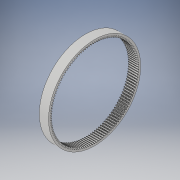
# Autodesk Inventor part: Component 21 (Hollow Wheel)
Saved by Autodesk Inventor 2018 (Build 220112000, 112)
## iProperties
Created: 2023-03-18
Part Number: Component 21 (Hollow Wheel)
Material: Generic
Document SubType Name: Modeling
Designer: Habib Mohamed
Density: 1 g/cm^3
Appearance: Default
Author: Habib Mohamed
Autodesk Inventor part; units mm, degrees
(part 1 of 2)
ref_plane "YZ Plane" through (0, 0, 0) normal (1, 0, 0) x (0, 1, 0)
ref_plane "XZ Plane" through (0, 0, 0) normal (0, 1, 0) x (-1, 0, 0)
ref_plane "XY Plane" through (0, 0, 0) normal (0, 0, 1) x (1, 0, 0)
sketch "Sketch1" plane through (0, 0, 0) normal (1, 0, 0) x (0, 1, 0)
  circle A0 centre (0, 0) radius 35
  line L0 (0, 0) -> (50.8877, 0) construction
  arc A1 (33.5687, 0.2221) -> (32.568, 0.5633) centre (30.706, -6.5366) ccw
  arc A2 (33.6297, 0.1304) -> (33.5687, 0.2221) centre (33.5297, 0.13) ccw
  arc A3 (32.4933, 0.658) -> (32.568, 0.5633) centre (32.5933, 0.66) ccw
  arc A4 (32.568, -0.5633) -> (33.5687, -0.2221) centre (30.706, 6.5366) ccw
  arc A5 (33.5687, -0.2221) -> (33.6297, -0.1304) centre (33.5297, -0.13) ccw
  arc A6 (32.568, -0.5633) -> (32.4933, -0.658) centre (32.5933, -0.66) ccw
  arc A7 (32.4252, 2.2033) -> (32.5043, 2.1123) centre (32.525, 2.2101) ccw
  arc A8 (33.5413, 1.3754) -> (33.5979, 1.4699) centre (33.498, 1.4656) ccw
  arc A9 (32.5579, 0.987) -> (33.5413, 1.3754) centre (30.3602, 7.9903) ccw
  arc A10 (32.5579, 0.987) -> (32.4878, 0.8889) centre (32.5878, 0.8916) ccw
  arc A11 (33.5202, 1.8191) -> (32.5043, 2.1123) centre (30.9823, -5.0682) ccw
  arc A12 (33.5855, 1.7304) -> (33.5202, 1.8191) centre (33.4856, 1.7253) ccw
  arc A13 (32.2837, 3.7437) -> (32.3669, 3.6565) centre (32.383, 3.7552) ccw
  arc A14 (33.4379, 2.9698) -> (33.4899, 3.0669) centre (33.3903, 3.0578) ccw
  arc A15 (32.474, 2.5351) -> (33.4379, 2.9698) centre (29.9456, 9.4258) ccw
  arc A16 (32.474, 2.5351) -> (32.4088, 2.4337) centre (32.5085, 2.4412) ccw
  arc A17 (33.3956, 3.412) -> (32.3669, 3.6565) centre (31.1883, -3.5883) ccw
  arc A18 (33.4651, 3.3265) -> (33.3956, 3.412) centre (33.3656, 3.3166) ccw
  arc A19 (32.069, 5.2756) -> (32.1563, 5.1924) centre (32.1676, 5.2918) ccw
  arc A20 (33.2587, 4.5575) -> (33.306, 4.657) centre (33.207, 4.6431) ccw
  arc A21 (32.3166, 4.0774) -> (33.2587, 4.5575) centre (29.4632, 10.84) ccw
  arc A22 (32.3166, 4.0774) -> (32.2562, 3.973) centre (32.3555, 3.9852) ccw
  arc A23 (33.1955, 4.9972) -> (32.1563, 5.1924) centre (31.3237, -2.1002) ccw
  arc A24 (33.2689, 4.9151) -> (33.1955, 4.9972) centre (33.17, 4.9005) ccw
  arc A25 (31.7816, 6.7955) -> (31.8728, 6.7166) centre (31.8794, 6.8164) ccw
  arc A26 (33.0041, 6.1349) -> (33.0467, 6.2364) centre (32.9484, 6.2179) ccw
  arc A27 (32.086, 5.6104) -> (33.0041, 6.1349) centre (28.9141, 12.2297) ccw
  arc A28 (32.086, 5.6104) -> (32.0307, 5.5033) centre (32.1292, 5.5203) ccw
  arc A29 (32.9201, 6.571) -> (31.8728, 6.7166) centre (31.3882, -0.6074) ccw
  arc A30 (32.9973, 6.4925) -> (32.9201, 6.571) centre (32.8992, 6.4732) ccw
  arc A31 (31.4223, 8.3) -> (31.5171, 8.2256) centre (31.519, 8.3256) ccw
  arc A32 (32.6749, 7.6983) -> (32.7125, 7.8018) centre (32.6152, 7.7786) ccw
  arc A33 (31.7827, 7.1308) -> (32.6749, 7.6983) centre (28.2994, 13.5916) ccw
  arc A34 (31.7827, 7.1308) -> (31.7325, 7.0212) centre (31.8302, 7.0428) ccw
  arc A35 (32.5701, 8.13) -> (31.5171, 8.2256) centre (31.3815, 0.8868) ccw
  arc A36 (32.651, 8.0552) -> (32.5701, 8.13) centre (32.5539, 8.0313) ccw
  arc A37 (30.9918, 9.7858) -> (31.09, 9.7159) centre (31.0871, 9.8159) ccw
  arc A38 (32.2715, 9.2443) -> (32.3042, 9.3495) centre (32.2082, 9.3217) ccw
  arc A39 (31.4074, 8.635) -> (32.2715, 9.2443) centre (27.6206, 14.9228) ccw
  arc A40 (31.4074, 8.635) -> (31.3625, 8.5231) centre (31.459, 8.5493) ccw
  arc A41 (32.1464, 9.6705) -> (31.09, 9.7159) centre (31.3038, 2.379) ccw
  arc A42 (32.2308, 9.5997) -> (32.1464, 9.6705) centre (32.1349, 9.5712) ccw
  arc A43 (30.491, 11.2493) -> (30.5925, 11.1842) centre (30.5848, 11.2839) ccw
  arc A44 (31.7951, 10.7694) -> (31.8228, 10.876) centre (31.7282, 10.8437) ccw
  arc A45 (30.961, 10.1196) -> (31.7951, 10.7694) centre (26.8793, 16.2201) ccw
  arc A46 (30.961, 10.1196) -> (30.9214, 10.0057) centre (31.0166, 10.0365) ccw
  arc A47 (31.6499, 11.1891) -> (30.5925, 11.1842) centre (31.1551, 3.8658) ccw
  arc A48 (31.7375, 11.1224) -> (31.6499, 11.1891) centre (31.6431, 11.0894) ccw
  arc A49 (29.9212, 12.6874) -> (30.0257, 12.6272) centre (30.0133, 12.7264) ccw
  arc A50 (31.2467, 12.2701) -> (31.2692, 12.3779) centre (31.1763, 12.3411) ccw
  arc A51 (30.4444, 11.5814) -> (31.2467, 12.2701) centre (26.0771, 17.4807) ccw
  arc A52 (30.4444, 11.5814) -> (30.4103, 11.4657) centre (30.5039, 11.501) ccw
  arc A53 (31.0816, 12.6824) -> (30.0257, 12.6272) centre (30.9359, 5.3439) ccw
  arc A54 (31.1723, 12.62) -> (31.0816, 12.6824) centre (31.0796, 12.5824) ccw
  arc A55 (29.2836, 14.0967) -> (29.3909, 14.0416) centre (29.3738, 14.1401) ccw
  arc A56 (30.6275, 13.743) -> (30.6449, 13.8517) centre (30.5537, 13.8105) ccw
  arc A57 (29.8588, 13.0168) -> (30.6275, 13.743) centre (25.2158, 18.7017) ccw
  arc A58 (29.8588, 13.0168) -> (29.8303, 12.8997) centre (29.9221, 12.9394) ccw
  arc A59 (30.443, 14.147) -> (29.3909, 14.0416) centre (30.6466, 6.8098) ccw
  arc A60 (30.5365, 14.0889) -> (30.443, 14.147) centre (30.4457, 14.047) ccw
  arc A61 (28.5797, 15.4741) -> (28.6894, 15.4242) centre (28.6677, 15.5218) ccw
  arc A62 (29.9389, 15.1847) -> (29.9511, 15.2941) centre (29.862, 15.2487) ccw
  arc A63 (29.2057, 14.4228) -> (29.9389, 15.1847) centre (24.2973, 19.8803) ccw
  arc A64 (29.2057, 14.4228) -> (29.1827, 14.3045) centre (29.2725, 14.3485) ccw
  arc A65 (29.7353, 15.5795) -> (28.6894, 15.4242) centre (30.2879, 8.2603) ccw
  arc A66 (29.8316, 15.5259) -> (29.7353, 15.5795) centre (29.7429, 15.4798) ccw
  arc A67 (27.8111, 16.8165) -> (27.923, 16.7718) centre (27.8966, 16.8682) ccw
  arc A68 (29.1824, 16.592) -> (29.1894, 16.702) centre (29.1026, 16.6523) ccw
  arc A69 (28.4863, 15.7962) -> (29.1824, 16.592) centre (23.3239, 21.0139) ccw
  arc A70 (28.4863, 15.7962) -> (28.469, 15.6768) centre (28.5566, 15.7251) ccw
  arc A71 (28.9603, 16.9767) -> (27.923, 16.7718) centre (29.8605, 9.6921) ccw
  arc A72 (29.059, 16.9278) -> (28.9603, 16.9767) centre (28.9726, 16.8775) ccw
  arc A73 (26.9794, 18.1207) -> (27.0934, 18.0814) centre (27.0624, 18.1765) ccw
  arc A74 (28.3599, 17.9618) -> (28.3616, 18.0719) centre (28.2773, 18.0182) ccw
  arc A75 (27.7024, 17.1337) -> (28.3599, 17.9618) centre (22.2976, 22.0999) ccw
  arc A76 (27.7024, 17.1337) -> (27.6909, 17.0137) centre (27.7761, 17.0661) ccw
  arc A77 (28.1198, 18.3355) -> (27.0934, 18.0814) centre (29.3655, 11.102) ccw
  arc A78 (28.2207, 18.2913) -> (28.1198, 18.3355) centre (28.1367, 18.2369) ccw
  arc A79 (26.0866, 19.384) -> (26.2023, 19.3501) centre (26.1669, 19.4436) ccw
  arc A80 (27.4731, 19.2909) -> (27.4696, 19.401) centre (27.3879, 19.3433) ccw
  arc A81 (26.8558, 18.4324) -> (27.4731, 19.2909) centre (21.2208, 23.1358) ccw
  arc A82 (26.8558, 18.4324) -> (26.85, 18.312) centre (26.9326, 18.3684) ccw
  arc A83 (27.2155, 19.6527) -> (26.2023, 19.3501) centre (28.804, 12.4866) ccw
  arc A84 (27.3184, 19.6134) -> (27.2155, 19.6527) centre (27.2371, 19.5551) ccw
  arc A85 (25.1348, 20.6033) -> (25.2519, 20.5749) centre (25.2121, 20.6666) ccw
  arc A86 (26.5241, 20.5763) -> (26.5154, 20.686) centre (26.4365, 20.6245) ccw
  arc A87 (25.9483, 19.6894) -> (26.5241, 20.5763) centre (20.0959, 24.1194) ccw
  arc A88 (25.9483, 19.6894) -> (25.9482, 19.5688) centre (26.0281, 19.6291) ccw
  arc A89 (26.2495, 20.9254) -> (25.2519, 20.5749) centre (28.1772, 13.8431) ccw
  arc A90 (26.3542, 20.891) -> (26.2495, 20.9254) centre (26.2758, 20.8289) ccw
  arc A91 (24.1259, 21.7759) -> (24.2444, 21.7532) centre (24.2002, 21.8429) ccw
  arc A92 (25.515, 21.815) -> (25.5011, 21.9243) centre (25.4252, 21.8591) ccw
  arc A93 (24.9821, 20.9018) -> (25.515, 21.815) centre (18.9255, 25.0482) ccw
  arc A94 (24.9821, 20.9018) -> (24.9877, 20.7813) centre (25.0646, 20.8453) ccw
  arc A95 (25.2241, 22.1507) -> (24.2444, 21.7532) centre (27.4867, 15.1681) ccw
  arc A96 (25.3303, 22.1213) -> (25.2241, 22.1507) centre (25.255, 22.0556) ccw
  arc A97 (23.0625, 22.8992) -> (23.1818, 22.8821) centre (23.1334, 22.9696) ccw
  arc A98 (24.4481, 23.0044) -> (24.429, 23.1128) centre (24.3563, 23.0441) ccw
  arc A99 (23.9592, 22.0668) -> (24.4481, 23.0044) centre (17.7122, 25.9204) ccw
  arc A100 (23.9592, 22.0668) -> (23.9706, 21.9468) centre (24.0443, 22.0143) ccw
  arc A101 (24.1416, 23.3258) -> (23.1818, 22.8821) centre (26.7338, 16.4588) ccw
  arc A102 (24.249, 23.3015) -> (24.1416, 23.3258) centre (24.1769, 23.2323) ccw
  arc A103 (21.9468, 23.9706) -> (22.0668, 23.9592) centre (22.0143, 24.0443) ccw
  arc A104 (23.3258, 24.1416) -> (23.3015, 24.249) centre (23.2323, 24.1769) ccw
  arc A105 (22.8821, 23.1818) -> (23.3258, 24.1416) centre (16.4588, 26.7338) ccw
  arc A106 (22.8821, 23.1818) -> (22.8992, 23.0625) centre (22.9696, 23.1334) ccw
  arc A107 (23.0044, 24.4481) -> (22.0668, 23.9592) centre (25.9204, 17.7122) ccw
  arc A108 (23.1128, 24.429) -> (23.0044, 24.4481) centre (23.0441, 24.3563) ccw
  arc A109 (20.7813, 24.9877) -> (20.9018, 24.9821) centre (20.8453, 25.0646) ccw
  arc A110 (22.1507, 25.2241) -> (22.1213, 25.3303) centre (22.0556, 25.255) ccw
  arc A111 (21.7532, 24.2444) -> (22.1507, 25.2241) centre (15.1681, 27.4867) ccw
  arc A112 (21.7532, 24.2444) -> (21.7759, 24.1259) centre (21.8429, 24.2002) ccw
  arc A113 (21.815, 25.515) -> (20.9018, 24.9821) centre (25.0482, 18.9255) ccw
  arc A114 (21.9243, 25.5011) -> (21.815, 25.515) centre (21.8591, 25.4252) ccw
  arc A115 (19.5688, 25.9482) -> (19.6894, 25.9483) centre (19.6291, 26.0281) ccw
  arc A116 (20.9254, 26.2495) -> (20.891, 26.3542) centre (20.8289, 26.2758) ccw
  arc A117 (20.5749, 25.2519) -> (20.9254, 26.2495) centre (13.8431, 28.1772) ccw
  arc A118 (20.5749, 25.2519) -> (20.6033, 25.1348) centre (20.6666, 25.2121) ccw
  arc A119 (20.5763, 26.5241) -> (19.6894, 25.9483) centre (24.1194, 20.0959) ccw
  arc A120 (20.686, 26.5154) -> (20.5763, 26.5241) centre (20.6245, 26.4365) ccw
  arc A121 (18.312, 26.85) -> (18.4324, 26.8558) centre (18.3684, 26.9326) ccw
  arc A122 (19.6527, 27.2155) -> (19.6134, 27.3184) centre (19.5551, 27.2371) ccw
  arc A123 (19.3501, 26.2023) -> (19.6527, 27.2155) centre (12.4866, 28.804) ccw
  arc A124 (19.3501, 26.2023) -> (19.384, 26.0866) centre (19.4436, 26.1669) ccw
  arc A125 (19.2909, 27.4731) -> (18.4324, 26.8558) centre (23.1358, 21.2208) ccw
  arc A126 (19.401, 27.4696) -> (19.2909, 27.4731) centre (19.3433, 27.3879) ccw
  arc A127 (17.0137, 27.6909) -> (17.1337, 27.7024) centre (17.0661, 27.7761) ccw
  arc A128 (18.3355, 28.1198) -> (18.2913, 28.2207) centre (18.2369, 28.1367) ccw
  arc A129 (18.0814, 27.0934) -> (18.3355, 28.1198) centre (11.102, 29.3655) ccw
  arc A130 (18.0814, 27.0934) -> (18.1207, 26.9794) centre (18.1765, 27.0624) ccw
  arc A131 (17.9618, 28.3599) -> (17.1337, 27.7024) centre (22.0999, 22.2976) ccw
  arc A132 (18.0719, 28.3616) -> (17.9618, 28.3599) centre (18.0182, 28.2773) ccw
  arc A133 (15.6768, 28.469) -> (15.7962, 28.4863) centre (15.7251, 28.5566) ccw
  arc A134 (16.9767, 28.9603) -> (16.9278, 29.059) centre (16.8775, 28.9726) ccw
  arc A135 (16.7718, 27.923) -> (16.9767, 28.9603) centre (9.6921, 29.8605) ccw
  arc A136 (16.7718, 27.923) -> (16.8165, 27.8111) centre (16.8682, 27.8966) ccw
  arc A137 (16.592, 29.1824) -> (15.7962, 28.4863) centre (21.0139, 23.3239) ccw
  arc A138 (16.702, 29.1894) -> (16.592, 29.1824) centre (16.6523, 29.1026) ccw
  arc A139 (14.3045, 29.1827) -> (14.4228, 29.2057) centre (14.3485, 29.2725) ccw
  arc A140 (15.5795, 29.7353) -> (15.5259, 29.8316) centre (15.4798, 29.7429) ccw
  arc A141 (15.4242, 28.6894) -> (15.5795, 29.7353) centre (8.2603, 30.2879) ccw
  arc A142 (15.4242, 28.6894) -> (15.4741, 28.5797) centre (15.5218, 28.6677) ccw
  arc A143 (15.1847, 29.9389) -> (14.4228, 29.2057) centre (19.8803, 24.2973) ccw
  arc A144 (15.2941, 29.9511) -> (15.1847, 29.9389) centre (15.2487, 29.862) ccw
  arc A145 (12.8997, 29.8303) -> (13.0168, 29.8588) centre (12.9394, 29.9221) ccw
  arc A146 (14.147, 30.443) -> (14.0889, 30.5365) centre (14.047, 30.4457) ccw
  arc A147 (14.0416, 29.3909) -> (14.147, 30.443) centre (6.8098, 30.6466) ccw
  arc A148 (14.0416, 29.3909) -> (14.0967, 29.2836) centre (14.1401, 29.3738) ccw
  arc A149 (13.743, 30.6275) -> (13.0168, 29.8588) centre (18.7017, 25.2158) ccw
  arc A150 (13.8517, 30.6449) -> (13.743, 30.6275) centre (13.8105, 30.5537) ccw
  arc A151 (11.4657, 30.4103) -> (11.5814, 30.4444) centre (11.501, 30.5039) ccw
  arc A152 (12.6824, 31.0816) -> (12.62, 31.1723) centre (12.5824, 31.0796) ccw
  arc A153 (12.6272, 30.0257) -> (12.6824, 31.0816) centre (5.3439, 30.9359) ccw
  arc A154 (12.6272, 30.0257) -> (12.6874, 29.9212) centre (12.7264, 30.0133) ccw
  arc A155 (12.2701, 31.2467) -> (11.5814, 30.4444) centre (17.4807, 26.0771) ccw
  arc A156 (12.3779, 31.2692) -> (12.2701, 31.2467) centre (12.3411, 31.1763) ccw
  arc A157 (10.0057, 30.9214) -> (10.1196, 30.961) centre (10.0365, 31.0166) ccw
  arc A158 (11.1891, 31.6499) -> (11.1224, 31.7375) centre (11.0894, 31.6431) ccw
  arc A159 (11.1842, 30.5925) -> (11.1891, 31.6499) centre (3.8658, 31.1551) ccw
  arc A160 (11.1842, 30.5925) -> (11.2493, 30.491) centre (11.2839, 30.5848) ccw
  arc A161 (10.7694, 31.7951) -> (10.1196, 30.961) centre (16.2201, 26.8793) ccw
  arc A162 (10.876, 31.8228) -> (10.7694, 31.7951) centre (10.8437, 31.7282) ccw
  arc A163 (8.5231, 31.3625) -> (8.635, 31.4074) centre (8.5493, 31.459) ccw
  arc A164 (9.6705, 32.1464) -> (9.5997, 32.2308) centre (9.5712, 32.1349) ccw
  arc A165 (9.7159, 31.09) -> (9.6705, 32.1464) centre (2.379, 31.3038) ccw
  arc A166 (9.7159, 31.09) -> (9.7858, 30.9918) centre (9.8159, 31.0871) ccw
  arc A167 (9.2443, 32.2715) -> (8.635, 31.4074) centre (14.9228, 27.6206) ccw
  arc A168 (9.3495, 32.3042) -> (9.2443, 32.2715) centre (9.3217, 32.2082) ccw
  arc A169 (7.0212, 31.7325) -> (7.1308, 31.7827) centre (7.0428, 31.8302) ccw
  arc A170 (8.13, 32.5701) -> (8.0552, 32.651) centre (8.0313, 32.5539) ccw
  arc A171 (8.2256, 31.5171) -> (8.13, 32.5701) centre (0.8868, 31.3815) ccw
  arc A172 (8.2256, 31.5171) -> (8.3, 31.4223) centre (8.3256, 31.519) ccw
  arc A173 (7.6983, 32.6749) -> (7.1308, 31.7827) centre (13.5916, 28.2994) ccw
  arc A174 (7.8018, 32.7125) -> (7.6983, 32.6749) centre (7.7786, 32.6152) ccw
  arc A175 (5.5033, 32.0307) -> (5.6104, 32.086) centre (5.5203, 32.1292) ccw
  arc A176 (6.571, 32.9201) -> (6.4925, 32.9973) centre (6.4732, 32.8992) ccw
  arc A177 (6.7166, 31.8728) -> (6.571, 32.9201) centre (-0.6074, 31.3882) ccw
  arc A178 (6.7166, 31.8728) -> (6.7955, 31.7816) centre (6.8164, 31.8794) ccw
  arc A179 (6.1349, 33.0041) -> (5.6104, 32.086) centre (12.2297, 28.9141) ccw
  arc A180 (6.2364, 33.0467) -> (6.1349, 33.0041) centre (6.2179, 32.9484) ccw
  arc A181 (3.973, 32.2562) -> (4.0774, 32.3166) centre (3.9852, 32.3555) ccw
  arc A182 (4.9972, 33.1955) -> (4.9151, 33.2689) centre (4.9005, 33.17) ccw
  arc A183 (5.1924, 32.1563) -> (4.9972, 33.1955) centre (-2.1002, 31.3237) ccw
  arc A184 (5.1924, 32.1563) -> (5.2756, 32.069) centre (5.2918, 32.1676) ccw
  arc A185 (4.5575, 33.2587) -> (4.0774, 32.3166) centre (10.84, 29.4632) ccw
  arc A186 (4.657, 33.306) -> (4.5575, 33.2587) centre (4.6431, 33.207) ccw
  arc A187 (2.4337, 32.4088) -> (2.5351, 32.474) centre (2.4412, 32.5085) ccw
  arc A188 (3.412, 33.3956) -> (3.3265, 33.4651) centre (3.3166, 33.3656) ccw
  arc A189 (3.6565, 32.3669) -> (3.412, 33.3956) centre (-3.5883, 31.1883) ccw
  arc A190 (3.6565, 32.3669) -> (3.7437, 32.2837) centre (3.7552, 32.383) ccw
  arc A191 (2.9698, 33.4379) -> (2.5351, 32.474) centre (9.4258, 29.9456) ccw
  arc A192 (3.0669, 33.4899) -> (2.9698, 33.4379) centre (3.0578, 33.3903) ccw
  arc A193 (0.8889, 32.4878) -> (0.987, 32.5579) centre (0.8916, 32.5878) ccw
  arc A194 (1.8191, 33.5202) -> (1.7304, 33.5855) centre (1.7253, 33.4856) ccw
  arc A195 (2.1123, 32.5043) -> (1.8191, 33.5202) centre (-5.0682, 30.9823) ccw
  arc A196 (2.1123, 32.5043) -> (2.2033, 32.4252) centre (2.2101, 32.525) ccw
  arc A197 (1.3754, 33.5413) -> (0.987, 32.5579) centre (7.9903, 30.3602) ccw
  arc A198 (1.4699, 33.5979) -> (1.3754, 33.5413) centre (1.4656, 33.498) ccw
  arc A199 (-0.658, 32.4933) -> (-0.5633, 32.568) centre (-0.66, 32.5933) ccw
  arc A200 (0.2221, 33.5687) -> (0.1304, 33.6297) centre (0.13, 33.5297) ccw
  arc A201 (0.5633, 32.568) -> (0.2221, 33.5687) centre (-6.5366, 30.706) ccw
  arc A202 (0.5633, 32.568) -> (0.658, 32.4933) centre (0.66, 32.5933) ccw
  arc A203 (-0.2221, 33.5687) -> (-0.5633, 32.568) centre (6.5366, 30.706) ccw
  arc A204 (-0.1304, 33.6297) -> (-0.2221, 33.5687) centre (-0.13, 33.5297) ccw
  arc A205 (-2.2033, 32.4252) -> (-2.1123, 32.5043) centre (-2.2101, 32.525) ccw
  arc A206 (-1.3754, 33.5413) -> (-1.4699, 33.5979) centre (-1.4656, 33.498) ccw
  arc A207 (-0.987, 32.5579) -> (-1.3754, 33.5413) centre (-7.9903, 30.3602) ccw
  arc A208 (-0.987, 32.5579) -> (-0.8889, 32.4878) centre (-0.8916, 32.5878) ccw
  arc A209 (-1.8191, 33.5202) -> (-2.1123, 32.5043) centre (5.0682, 30.9823) ccw
  arc A210 (-1.7304, 33.5855) -> (-1.8191, 33.5202) centre (-1.7253, 33.4856) ccw
  arc A211 (-3.7437, 32.2837) -> (-3.6565, 32.3669) centre (-3.7552, 32.383) ccw
  arc A212 (-2.9698, 33.4379) -> (-3.0669, 33.4899) centre (-3.0578, 33.3903) ccw
  arc A213 (-2.5351, 32.474) -> (-2.9698, 33.4379) centre (-9.4258, 29.9456) ccw
  arc A214 (-2.5351, 32.474) -> (-2.4337, 32.4088) centre (-2.4412, 32.5085) ccw
  arc A215 (-3.412, 33.3956) -> (-3.6565, 32.3669) centre (3.5883, 31.1883) ccw
  arc A216 (-3.3265, 33.4651) -> (-3.412, 33.3956) centre (-3.3166, 33.3656) ccw
  arc A217 (-5.2756, 32.069) -> (-5.1924, 32.1563) centre (-5.2918, 32.1676) ccw
  arc A218 (-4.5575, 33.2587) -> (-4.657, 33.306) centre (-4.6431, 33.207) ccw
  arc A219 (-4.0774, 32.3166) -> (-4.5575, 33.2587) centre (-10.84, 29.4632) ccw
  arc A220 (-4.0774, 32.3166) -> (-3.973, 32.2562) centre (-3.9852, 32.3555) ccw
  arc A221 (-4.9972, 33.1955) -> (-5.1924, 32.1563) centre (2.1002, 31.3237) ccw
  arc A222 (-4.9151, 33.2689) -> (-4.9972, 33.1955) centre (-4.9005, 33.17) ccw
  arc A223 (-6.7955, 31.7816) -> (-6.7166, 31.8728) centre (-6.8164, 31.8794) ccw
  arc A224 (-6.1349, 33.0041) -> (-6.2364, 33.0467) centre (-6.2179, 32.9484) ccw
  arc A225 (-5.6104, 32.086) -> (-6.1349, 33.0041) centre (-12.2297, 28.9141) ccw
  arc A226 (-5.6104, 32.086) -> (-5.5033, 32.0307) centre (-5.5203, 32.1292) ccw
  arc A227 (-6.571, 32.9201) -> (-6.7166, 31.8728) centre (0.6074, 31.3882) ccw
  arc A228 (-6.4925, 32.9973) -> (-6.571, 32.9201) centre (-6.4732, 32.8992) ccw
  arc A229 (-8.3, 31.4223) -> (-8.2256, 31.5171) centre (-8.3256, 31.519) ccw
  arc A230 (-7.6983, 32.6749) -> (-7.8018, 32.7125) centre (-7.7786, 32.6152) ccw
  arc A231 (-7.1308, 31.7827) -> (-7.6983, 32.6749) centre (-13.5916, 28.2994) ccw
  arc A232 (-7.1308, 31.7827) -> (-7.0212, 31.7325) centre (-7.0428, 31.8302) ccw
  arc A233 (-8.13, 32.5701) -> (-8.2256, 31.5171) centre (-0.8868, 31.3815) ccw
  arc A234 (-8.0552, 32.651) -> (-8.13, 32.5701) centre (-8.0313, 32.5539) ccw
  arc A235 (-9.7858, 30.9918) -> (-9.7159, 31.09) centre (-9.8159, 31.0871) ccw
  arc A236 (-9.2443, 32.2715) -> (-9.3495, 32.3042) centre (-9.3217, 32.2082) ccw
  arc A237 (-8.635, 31.4074) -> (-9.2443, 32.2715) centre (-14.9228, 27.6206) ccw
  arc A238 (-8.635, 31.4074) -> (-8.5231, 31.3625) centre (-8.5493, 31.459) ccw
  arc A239 (-9.6705, 32.1464) -> (-9.7159, 31.09) centre (-2.379, 31.3038) ccw
  arc A240 (-9.5997, 32.2308) -> (-9.6705, 32.1464) centre (-9.5712, 32.1349) ccw
  arc A241 (-11.2493, 30.491) -> (-11.1842, 30.5925) centre (-11.2839, 30.5848) ccw
  arc A242 (-10.7694, 31.7951) -> (-10.876, 31.8228) centre (-10.8437, 31.7282) ccw
  arc A243 (-10.1196, 30.961) -> (-10.7694, 31.7951) centre (-16.2201, 26.8793) ccw
  arc A244 (-10.1196, 30.961) -> (-10.0057, 30.9214) centre (-10.0365, 31.0166) ccw
  arc A245 (-11.1891, 31.6499) -> (-11.1842, 30.5925) centre (-3.8658, 31.1551) ccw
  arc A246 (-11.1224, 31.7375) -> (-11.1891, 31.6499) centre (-11.0894, 31.6431) ccw
  arc A247 (-12.6874, 29.9212) -> (-12.6272, 30.0257) centre (-12.7264, 30.0133) ccw
  arc A248 (-12.2701, 31.2467) -> (-12.3779, 31.2692) centre (-12.3411, 31.1763) ccw
  arc A249 (-11.5814, 30.4444) -> (-12.2701, 31.2467) centre (-17.4807, 26.0771) ccw
  arc A250 (-11.5814, 30.4444) -> (-11.4657, 30.4103) centre (-11.501, 30.5039) ccw
  arc A251 (-12.6824, 31.0816) -> (-12.6272, 30.0257) centre (-5.3439, 30.9359) ccw
  arc A252 (-12.62, 31.1723) -> (-12.6824, 31.0816) centre (-12.5824, 31.0796) ccw
  arc A253 (-14.0967, 29.2836) -> (-14.0416, 29.3909) centre (-14.1401, 29.3738) ccw
  arc A254 (-13.743, 30.6275) -> (-13.8517, 30.6449) centre (-13.8105, 30.5537) ccw
  arc A255 (-13.0168, 29.8588) -> (-13.743, 30.6275) centre (-18.7017, 25.2158) ccw
  arc A256 (-13.0168, 29.8588) -> (-12.8997, 29.8303) centre (-12.9394, 29.9221) ccw
  arc A257 (-14.147, 30.443) -> (-14.0416, 29.3909) centre (-6.8098, 30.6466) ccw
  arc A258 (-14.0889, 30.5365) -> (-14.147, 30.443) centre (-14.047, 30.4457) ccw
  arc A259 (-15.4741, 28.5797) -> (-15.4242, 28.6894) centre (-15.5218, 28.6677) ccw
  arc A260 (-15.1847, 29.9389) -> (-15.2941, 29.9511) centre (-15.2487, 29.862) ccw
  arc A261 (-14.4228, 29.2057) -> (-15.1847, 29.9389) centre (-19.8803, 24.2973) ccw
  arc A262 (-14.4228, 29.2057) -> (-14.3045, 29.1827) centre (-14.3485, 29.2725) ccw
  arc A263 (-15.5795, 29.7353) -> (-15.4242, 28.6894) centre (-8.2603, 30.2879) ccw
  arc A264 (-15.5259, 29.8316) -> (-15.5795, 29.7353) centre (-15.4798, 29.7429) ccw
  arc A265 (-16.8165, 27.8111) -> (-16.7718, 27.923) centre (-16.8682, 27.8966) ccw
  arc A266 (-16.592, 29.1824) -> (-16.702, 29.1894) centre (-16.6523, 29.1026) ccw
  arc A267 (-15.7962, 28.4863) -> (-16.592, 29.1824) centre (-21.0139, 23.3239) ccw
  arc A268 (-15.7962, 28.4863) -> (-15.6768, 28.469) centre (-15.7251, 28.5566) ccw
  arc A269 (-16.9767, 28.9603) -> (-16.7718, 27.923) centre (-9.6921, 29.8605) ccw
  arc A270 (-16.9278, 29.059) -> (-16.9767, 28.9603) centre (-16.8775, 28.9726) ccw
  arc A271 (-18.1207, 26.9794) -> (-18.0814, 27.0934) centre (-18.1765, 27.0624) ccw
  arc A272 (-17.9618, 28.3599) -> (-18.0719, 28.3616) centre (-18.0182, 28.2773) ccw
  arc A273 (-17.1337, 27.7024) -> (-17.9618, 28.3599) centre (-22.0999, 22.2976) ccw
  arc A274 (-17.1337, 27.7024) -> (-17.0137, 27.6909) centre (-17.0661, 27.7761) ccw
  arc A275 (-18.3355, 28.1198) -> (-18.0814, 27.0934) centre (-11.102, 29.3655) ccw
  arc A276 (-18.2913, 28.2207) -> (-18.3355, 28.1198) centre (-18.2369, 28.1367) ccw
  arc A277 (-19.384, 26.0866) -> (-19.3501, 26.2023) centre (-19.4436, 26.1669) ccw
  arc A278 (-19.2909, 27.4731) -> (-19.401, 27.4696) centre (-19.3433, 27.3879) ccw
  arc A279 (-18.4324, 26.8558) -> (-19.2909, 27.4731) centre (-23.1358, 21.2208) ccw
  arc A280 (-18.4324, 26.8558) -> (-18.312, 26.85) centre (-18.3684, 26.9326) ccw
  arc A281 (-19.6527, 27.2155) -> (-19.3501, 26.2023) centre (-12.4866, 28.804) ccw
  arc A282 (-19.6134, 27.3184) -> (-19.6527, 27.2155) centre (-19.5551, 27.2371) ccw
  arc A283 (-20.6033, 25.1348) -> (-20.5749, 25.2519) centre (-20.6666, 25.2121) ccw
  arc A284 (-20.5763, 26.5241) -> (-20.686, 26.5154) centre (-20.6245, 26.4365) ccw
  arc A285 (-19.6894, 25.9483) -> (-20.5763, 26.5241) centre (-24.1194, 20.0959) ccw
  arc A286 (-19.6894, 25.9483) -> (-19.5688, 25.9482) centre (-19.6291, 26.0281) ccw
  arc A287 (-20.9254, 26.2495) -> (-20.5749, 25.2519) centre (-13.8431, 28.1772) ccw
  arc A288 (-20.891, 26.3542) -> (-20.9254, 26.2495) centre (-20.8289, 26.2758) ccw
  arc A289 (-21.7759, 24.1259) -> (-21.7532, 24.2444) centre (-21.8429, 24.2002) ccw
  arc A290 (-21.815, 25.515) -> (-21.9243, 25.5011) centre (-21.8591, 25.4252) ccw
  arc A291 (-20.9018, 24.9821) -> (-21.815, 25.515) centre (-25.0482, 18.9255) ccw
  arc A292 (-20.9018, 24.9821) -> (-20.7813, 24.9877) centre (-20.8453, 25.0646) ccw
  arc A293 (-22.1507, 25.2241) -> (-21.7532, 24.2444) centre (-15.1681, 27.4867) ccw
  arc A294 (-22.1213, 25.3303) -> (-22.1507, 25.2241) centre (-22.0556, 25.255) ccw
  arc A295 (-22.8992, 23.0625) -> (-22.8821, 23.1818) centre (-22.9696, 23.1334) ccw
  arc A296 (-23.0044, 24.4481) -> (-23.1128, 24.429) centre (-23.0441, 24.3563) ccw
  arc A297 (-22.0668, 23.9592) -> (-23.0044, 24.4481) centre (-25.9204, 17.7122) ccw
  arc A298 (-22.0668, 23.9592) -> (-21.9468, 23.9706) centre (-22.0143, 24.0443) ccw
  arc A299 (-23.3258, 24.1416) -> (-22.8821, 23.1818) centre (-16.4588, 26.7338) ccw
  arc A300 (-23.3015, 24.249) -> (-23.3258, 24.1416) centre (-23.2323, 24.1769) ccw
  arc A301 (-23.9706, 21.9468) -> (-23.9592, 22.0668) centre (-24.0443, 22.0143) ccw
  arc A302 (-24.1416, 23.3258) -> (-24.249, 23.3015) centre (-24.1769, 23.2323) ccw
  arc A303 (-23.1818, 22.8821) -> (-24.1416, 23.3258) centre (-26.7338, 16.4588) ccw
  arc A304 (-23.1818, 22.8821) -> (-23.0625, 22.8992) centre (-23.1334, 22.9696) ccw
  arc A305 (-24.4481, 23.0044) -> (-23.9592, 22.0668) centre (-17.7122, 25.9204) ccw
  arc A306 (-24.429, 23.1128) -> (-24.4481, 23.0044) centre (-24.3563, 23.0441) ccw
  arc A307 (-24.9877, 20.7813) -> (-24.9821, 20.9018) centre (-25.0646, 20.8453) ccw
  arc A308 (-25.2241, 22.1507) -> (-25.3303, 22.1213) centre (-25.255, 22.0556) ccw
  arc A309 (-24.2444, 21.7532) -> (-25.2241, 22.1507) centre (-27.4867, 15.1681) ccw
  arc A310 (-24.2444, 21.7532) -> (-24.1259, 21.7759) centre (-24.2002, 21.8429) ccw
  arc A311 (-25.515, 21.815) -> (-24.9821, 20.9018) centre (-18.9255, 25.0482) ccw
  arc A312 (-25.5011, 21.9243) -> (-25.515, 21.815) centre (-25.4252, 21.8591) ccw
  arc A313 (-25.9482, 19.5688) -> (-25.9483, 19.6894) centre (-26.0281, 19.6291) ccw
  arc A314 (-26.2495, 20.9254) -> (-26.3542, 20.891) centre (-26.2758, 20.8289) ccw
  arc A315 (-25.2519, 20.5749) -> (-26.2495, 20.9254) centre (-28.1772, 13.8431) ccw
  arc A316 (-25.2519, 20.5749) -> (-25.1348, 20.6033) centre (-25.2121, 20.6666) ccw
  arc A317 (-26.5241, 20.5763) -> (-25.9483, 19.6894) centre (-20.0959, 24.1194) ccw
  arc A318 (-26.5154, 20.686) -> (-26.5241, 20.5763) centre (-26.4365, 20.6245) ccw
  arc A319 (-26.85, 18.312) -> (-26.8558, 18.4324) centre (-26.9326, 18.3684) ccw
  arc A320 (-27.2155, 19.6527) -> (-27.3184, 19.6134) centre (-27.2371, 19.5551) ccw
  arc A321 (-26.2023, 19.3501) -> (-27.2155, 19.6527) centre (-28.804, 12.4866) ccw
  arc A322 (-26.2023, 19.3501) -> (-26.0866, 19.384) centre (-26.1669, 19.4436) ccw
  arc A323 (-27.4731, 19.2909) -> (-26.8558, 18.4324) centre (-21.2208, 23.1358) ccw
  arc A324 (-27.4696, 19.401) -> (-27.4731, 19.2909) centre (-27.3879, 19.3433) ccw
  arc A325 (-27.6909, 17.0137) -> (-27.7024, 17.1337) centre (-27.7761, 17.0661) ccw
  arc A326 (-28.1198, 18.3355) -> (-28.2207, 18.2913) centre (-28.1367, 18.2369) ccw
  arc A327 (-27.0934, 18.0814) -> (-28.1198, 18.3355) centre (-29.3655, 11.102) ccw
  arc A328 (-27.0934, 18.0814) -> (-26.9794, 18.1207) centre (-27.0624, 18.1765) ccw
  arc A329 (-28.3599, 17.9618) -> (-27.7024, 17.1337) centre (-22.2976, 22.0999) ccw
  arc A330 (-28.3616, 18.0719) -> (-28.3599, 17.9618) centre (-28.2773, 18.0182) ccw
  arc A331 (-28.469, 15.6768) -> (-28.4863, 15.7962) centre (-28.5566, 15.7251) ccw
  arc A332 (-28.9603, 16.9767) -> (-29.059, 16.9278) centre (-28.9726, 16.8775) ccw
  arc A333 (-27.923, 16.7718) -> (-28.9603, 16.9767) centre (-29.8605, 9.6921) ccw
  arc A334 (-27.923, 16.7718) -> (-27.8111, 16.8165) centre (-27.8966, 16.8682) ccw
  arc A335 (-29.1824, 16.592) -> (-28.4863, 15.7962) centre (-23.3239, 21.0139) ccw
  arc A336 (-29.1894, 16.702) -> (-29.1824, 16.592) centre (-29.1026, 16.6523) ccw
  arc A337 (-29.1827, 14.3045) -> (-29.2057, 14.4228) centre (-29.2725, 14.3485) ccw
  arc A338 (-29.7353, 15.5795) -> (-29.8316, 15.5259) centre (-29.7429, 15.4798) ccw
  arc A339 (-28.6894, 15.4242) -> (-29.7353, 15.5795) centre (-30.2879, 8.2603) ccw
  arc A340 (-28.6894, 15.4242) -> (-28.5797, 15.4741) centre (-28.6677, 15.5218) ccw
  arc A341 (-29.9389, 15.1847) -> (-29.2057, 14.4228) centre (-24.2973, 19.8803) ccw
  arc A342 (-29.9511, 15.2941) -> (-29.9389, 15.1847) centre (-29.862, 15.2487) ccw
  arc A343 (-29.8303, 12.8997) -> (-29.8588, 13.0168) centre (-29.9221, 12.9394) ccw
  arc A344 (-30.443, 14.147) -> (-30.5365, 14.0889) centre (-30.4457, 14.047) ccw
  arc A345 (-29.3909, 14.0416) -> (-30.443, 14.147) centre (-30.6466, 6.8098) ccw
  arc A346 (-29.3909, 14.0416) -> (-29.2836, 14.0967) centre (-29.3738, 14.1401) ccw
  arc A347 (-30.6275, 13.743) -> (-29.8588, 13.0168) centre (-25.2158, 18.7017) ccw
  arc A348 (-30.6449, 13.8517) -> (-30.6275, 13.743) centre (-30.5537, 13.8105) ccw
  arc A349 (-30.4103, 11.4657) -> (-30.4444, 11.5814) centre (-30.5039, 11.501) ccw
  arc A350 (-31.0816, 12.6824) -> (-31.1723, 12.62) centre (-31.0796, 12.5824) ccw
  arc A351 (-30.0257, 12.6272) -> (-31.0816, 12.6824) centre (-30.9359, 5.3439) ccw
  arc A352 (-30.0257, 12.6272) -> (-29.9212, 12.6874) centre (-30.0133, 12.7264) ccw
  arc A353 (-31.2467, 12.2701) -> (-30.4444, 11.5814) centre (-26.0771, 17.4807) ccw
  arc A354 (-31.2692, 12.3779) -> (-31.2467, 12.2701) centre (-31.1763, 12.3411) ccw
  arc A355 (-30.9214, 10.0057) -> (-30.961, 10.1196) centre (-31.0166, 10.0365) ccw
  arc A356 (-31.6499, 11.1891) -> (-31.7375, 11.1224) centre (-31.6431, 11.0894) ccw
  arc A357 (-30.5925, 11.1842) -> (-31.6499, 11.1891) centre (-31.1551, 3.8658) ccw
  arc A358 (-30.5925, 11.1842) -> (-30.491, 11.2493) centre (-30.5848, 11.2839) ccw
  arc A359 (-31.7951, 10.7694) -> (-30.961, 10.1196) centre (-26.8793, 16.2201) ccw
  arc A360 (-31.8228, 10.876) -> (-31.7951, 10.7694) centre (-31.7282, 10.8437) ccw
  arc A361 (-31.3625, 8.5231) -> (-31.4074, 8.635) centre (-31.459, 8.5493) ccw
  arc A362 (-32.1464, 9.6705) -> (-32.2308, 9.5997) centre (-32.1349, 9.5712) ccw
  arc A363 (-31.09, 9.7159) -> (-32.1464, 9.6705) centre (-31.3038, 2.379) ccw
  arc A364 (-31.09, 9.7159) -> (-30.9918, 9.7858) centre (-31.0871, 9.8159) ccw
  arc A365 (-32.2715, 9.2443) -> (-31.4074, 8.635) centre (-27.6206, 14.9228) ccw
  arc A366 (-32.3042, 9.3495) -> (-32.2715, 9.2443) centre (-32.2082, 9.3217) ccw
  arc A367 (-31.7325, 7.0212) -> (-31.7827, 7.1308) centre (-31.8302, 7.0428) ccw
  arc A368 (-32.5701, 8.13) -> (-32.651, 8.0552) centre (-32.5539, 8.0313) ccw
  arc A369 (-31.5171, 8.2256) -> (-32.5701, 8.13) centre (-31.3815, 0.8868) ccw
  arc A370 (-31.5171, 8.2256) -> (-31.4223, 8.3) centre (-31.519, 8.3256) ccw
  arc A371 (-32.6749, 7.6983) -> (-31.7827, 7.1308) centre (-28.2994, 13.5916) ccw
  arc A372 (-32.7125, 7.8018) -> (-32.6749, 7.6983) centre (-32.6152, 7.7786) ccw
  arc A373 (-32.0307, 5.5033) -> (-32.086, 5.6104) centre (-32.1292, 5.5203) ccw
  arc A374 (-32.9201, 6.571) -> (-32.9973, 6.4925) centre (-32.8992, 6.4732) ccw
  arc A375 (-31.8728, 6.7166) -> (-32.9201, 6.571) centre (-31.3882, -0.6074) ccw
  arc A376 (-31.8728, 6.7166) -> (-31.7816, 6.7955) centre (-31.8794, 6.8164) ccw
  arc A377 (-33.0041, 6.1349) -> (-32.086, 5.6104) centre (-28.9141, 12.2297) ccw
  arc A378 (-33.0467, 6.2364) -> (-33.0041, 6.1349) centre (-32.9484, 6.2179) ccw
  arc A379 (-32.2562, 3.973) -> (-32.3166, 4.0774) centre (-32.3555, 3.9852) ccw
  arc A380 (-33.1955, 4.9972) -> (-33.2689, 4.9151) centre (-33.17, 4.9005) ccw
  arc A381 (-32.1563, 5.1924) -> (-33.1955, 4.9972) centre (-31.3237, -2.1002) ccw
  arc A382 (-32.1563, 5.1924) -> (-32.069, 5.2756) centre (-32.1676, 5.2918) ccw
  arc A383 (-33.2587, 4.5575) -> (-32.3166, 4.0774) centre (-29.4632, 10.84) ccw
  arc A384 (-33.306, 4.657) -> (-33.2587, 4.5575) centre (-33.207, 4.6431) ccw
  arc A385 (-32.4088, 2.4337) -> (-32.474, 2.5351) centre (-32.5085, 2.4412) ccw
  arc A386 (-33.3956, 3.412) -> (-33.4651, 3.3265) centre (-33.3656, 3.3166) ccw
  arc A387 (-32.3669, 3.6565) -> (-33.3956, 3.412) centre (-31.1883, -3.5883) ccw
  arc A388 (-32.3669, 3.6565) -> (-32.2837, 3.7437) centre (-32.383, 3.7552) ccw
  arc A389 (-33.4379, 2.9698) -> (-32.474, 2.5351) centre (-29.9456, 9.4258) ccw
  arc A390 (-33.4899, 3.0669) -> (-33.4379, 2.9698) centre (-33.3903, 3.0578) ccw
  arc A391 (-32.4878, 0.8889) -> (-32.5579, 0.987) centre (-32.5878, 0.8916) ccw
  arc A392 (-33.5202, 1.8191) -> (-33.5855, 1.7304) centre (-33.4856, 1.7253) ccw
  arc A393 (-32.5043, 2.1123) -> (-33.5202, 1.8191) centre (-30.9823, -5.0682) ccw
  arc A394 (-32.5043, 2.1123) -> (-32.4252, 2.2033) centre (-32.525, 2.2101) ccw
  arc A395 (-33.5413, 1.3754) -> (-32.5579, 0.987) centre (-30.3602, 7.9903) ccw
  arc A396 (-33.5979, 1.4699) -> (-33.5413, 1.3754) centre (-33.498, 1.4656) ccw
  arc A397 (-32.4933, -0.658) -> (-32.568, -0.5633) centre (-32.5933, -0.66) ccw
  arc A398 (-33.5687, 0.2221) -> (-33.6297, 0.1304) centre (-33.5297, 0.13) ccw
  arc A399 (-32.568, 0.5633) -> (-33.5687, 0.2221) centre (-30.706, -6.5366) ccw
  arc A400 (-32.568, 0.5633) -> (-32.4933, 0.658) centre (-32.5933, 0.66) ccw
  arc A401 (-33.5687, -0.2221) -> (-32.568, -0.5633) centre (-30.706, 6.5366) ccw
  arc A402 (-33.6297, -0.1304) -> (-33.5687, -0.2221) centre (-33.5297, -0.13) ccw
  arc A403 (-32.4252, -2.2033) -> (-32.5043, -2.1123) centre (-32.525, -2.2101) ccw
  arc A404 (-33.5413, -1.3754) -> (-33.5979, -1.4699) centre (-33.498, -1.4656) ccw
  arc A405 (-32.5579, -0.987) -> (-33.5413, -1.3754) centre (-30.3602, -7.9903) ccw
  arc A406 (-32.5579, -0.987) -> (-32.4878, -0.8889) centre (-32.5878, -0.8916) ccw
  arc A407 (-33.5202, -1.8191) -> (-32.5043, -2.1123) centre (-30.9823, 5.0682) ccw
  arc A408 (-33.5855, -1.7304) -> (-33.5202, -1.8191) centre (-33.4856, -1.7253) ccw
  arc A409 (-32.2837, -3.7437) -> (-32.3669, -3.6565) centre (-32.383, -3.7552) ccw
  arc A410 (-33.4379, -2.9698) -> (-33.4899, -3.0669) centre (-33.3903, -3.0578) ccw
  arc A411 (-32.474, -2.5351) -> (-33.4379, -2.9698) centre (-29.9456, -9.4258) ccw
  arc A412 (-32.474, -2.5351) -> (-32.4088, -2.4337) centre (-32.5085, -2.4412) ccw
  arc A413 (-33.3956, -3.412) -> (-32.3669, -3.6565) centre (-31.1883, 3.5883) ccw
  arc A414 (-33.4651, -3.3265) -> (-33.3956, -3.412) centre (-33.3656, -3.3166) ccw
  arc A415 (-32.069, -5.2756) -> (-32.1563, -5.1924) centre (-32.1676, -5.2918) ccw
  arc A416 (-33.2587, -4.5575) -> (-33.306, -4.657) centre (-33.207, -4.6431) ccw
  arc A417 (-32.3166, -4.0774) -> (-33.2587, -4.5575) centre (-29.4632, -10.84) ccw
  arc A418 (-32.3166, -4.0774) -> (-32.2562, -3.973) centre (-32.3555, -3.9852) ccw
  arc A419 (-33.1955, -4.9972) -> (-32.1563, -5.1924) centre (-31.3237, 2.1002) ccw
  arc A420 (-33.2689, -4.9151) -> (-33.1955, -4.9972) centre (-33.17, -4.9005) ccw
  arc A421 (-31.7816, -6.7955) -> (-31.8728, -6.7166) centre (-31.8794, -6.8164) ccw
  arc A422 (-33.0041, -6.1349) -> (-33.0467, -6.2364) centre (-32.9484, -6.2179) ccw
  arc A423 (-32.086, -5.6104) -> (-33.0041, -6.1349) centre (-28.9141, -12.2297) ccw
  arc A424 (-32.086, -5.6104) -> (-32.0307, -5.5033) centre (-32.1292, -5.5203) ccw
  arc A425 (-32.9201, -6.571) -> (-31.8728, -6.7166) centre (-31.3882, 0.6074) ccw
  arc A426 (-32.9973, -6.4925) -> (-32.9201, -6.571) centre (-32.8992, -6.4732) ccw
  arc A427 (-31.4223, -8.3) -> (-31.5171, -8.2256) centre (-31.519, -8.3256) ccw
  arc A428 (-32.6749, -7.6983) -> (-32.7125, -7.8018) centre (-32.6152, -7.7786) ccw
  arc A429 (-31.7827, -7.1308) -> (-32.6749, -7.6983) centre (-28.2994, -13.5916) ccw
  arc A430 (-31.7827, -7.1308) -> (-31.7325, -7.0212) centre (-31.8302, -7.0428) ccw
  arc A431 (-32.5701, -8.13) -> (-31.5171, -8.2256) centre (-31.3815, -0.8868) ccw
  arc A432 (-32.651, -8.0552) -> (-32.5701, -8.13) centre (-32.5539, -8.0313) ccw
  arc A433 (-30.9918, -9.7858) -> (-31.09, -9.7159) centre (-31.0871, -9.8159) ccw
  arc A434 (-32.2715, -9.2443) -> (-32.3042, -9.3495) centre (-32.2082, -9.3217) ccw
  arc A435 (-31.4074, -8.635) -> (-32.2715, -9.2443) centre (-27.6206, -14.9228) ccw
  arc A436 (-31.4074, -8.635) -> (-31.3625, -8.5231) centre (-31.459, -8.5493) ccw
  arc A437 (-32.1464, -9.6705) -> (-31.09, -9.7159) centre (-31.3038, -2.379) ccw
  arc A438 (-32.2308, -9.5997) -> (-32.1464, -9.6705) centre (-32.1349, -9.5712) ccw
  arc A439 (-30.491, -11.2493) -> (-30.5925, -11.1842) centre (-30.5848, -11.2839) ccw
  arc A440 (-31.7951, -10.7694) -> (-31.8228, -10.876) centre (-31.7282, -10.8437) ccw
  arc A441 (-30.961, -10.1196) -> (-31.7951, -10.7694) centre (-26.8793, -16.2201) ccw
  arc A442 (-30.961, -10.1196) -> (-30.9214, -10.0057) centre (-31.0166, -10.0365) ccw
  arc A443 (-31.6499, -11.1891) -> (-30.5925, -11.1842) centre (-31.1551, -3.8658) ccw
  arc A444 (-31.7375, -11.1224) -> (-31.6499, -11.1891) centre (-31.6431, -11.0894) ccw
  arc A445 (-29.9212, -12.6874) -> (-30.0257, -12.6272) centre (-30.0133, -12.7264) ccw
  arc A446 (-31.2467, -12.2701) -> (-31.2692, -12.3779) centre (-31.1763, -12.3411) ccw
  arc A447 (-30.4444, -11.5814) -> (-31.2467, -12.2701) centre (-26.0771, -17.4807) ccw
  arc A448 (-30.4444, -11.5814) -> (-30.4103, -11.4657) centre (-30.5039, -11.501) ccw
  arc A449 (-31.0816, -12.6824) -> (-30.0257, -12.6272) centre (-30.9359, -5.3439) ccw
  arc A450 (-31.1723, -12.62) -> (-31.0816, -12.6824) centre (-31.0796, -12.5824) ccw
  arc A451 (-29.2836, -14.0967) -> (-29.3909, -14.0416) centre (-29.3738, -14.1401) ccw
  arc A452 (-30.6275, -13.743) -> (-30.6449, -13.8517) centre (-30.5537, -13.8105) ccw
  arc A453 (-29.8588, -13.0168) -> (-30.6275, -13.743) centre (-25.2158, -18.7017) ccw
  arc A454 (-29.8588, -13.0168) -> (-29.8303, -12.8997) centre (-29.9221, -12.9394) ccw
  arc A455 (-30.443, -14.147) -> (-29.3909, -14.0416) centre (-30.6466, -6.8098) ccw
  arc A456 (-30.5365, -14.0889) -> (-30.443, -14.147) centre (-30.4457, -14.047) ccw
  arc A457 (-28.5797, -15.4741) -> (-28.6894, -15.4242) centre (-28.6677, -15.5218) ccw
  arc A458 (-29.9389, -15.1847) -> (-29.9511, -15.2941) centre (-29.862, -15.2487) ccw
  arc A459 (-29.2057, -14.4228) -> (-29.9389, -15.1847) centre (-24.2973, -19.8803) ccw
  arc A460 (-29.2057, -14.4228) -> (-29.1827, -14.3045) centre (-29.2725, -14.3485) ccw
  arc A461 (-29.7353, -15.5795) -> (-28.6894, -15.4242) centre (-30.2879, -8.2603) ccw
  arc A462 (-29.8316, -15.5259) -> (-29.7353, -15.5795) centre (-29.7429, -15.4798) ccw
  arc A463 (-27.8111, -16.8165) -> (-27.923, -16.7718) centre (-27.8966, -16.8682) ccw
  arc A464 (-29.1824, -16.592) -> (-29.1894, -16.702) centre (-29.1026, -16.6523) ccw
  arc A465 (-28.4863, -15.7962) -> (-29.1824, -16.592) centre (-23.3239, -21.0139) ccw
  arc A466 (-28.4863, -15.7962) -> (-28.469, -15.6768) centre (-28.5566, -15.7251) ccw
  arc A467 (-28.9603, -16.9767) -> (-27.923, -16.7718) centre (-29.8605, -9.6921) ccw
  arc A468 (-29.059, -16.9278) -> (-28.9603, -16.9767) centre (-28.9726, -16.8775) ccw
  arc A469 (-26.9794, -18.1207) -> (-27.0934, -18.0814) centre (-27.0624, -18.1765) ccw
  arc A470 (-28.3599, -17.9618) -> (-28.3616, -18.0719) centre (-28.2773, -18.0182) ccw
  arc A471 (-27.7024, -17.1337) -> (-28.3599, -17.9618) centre (-22.2976, -22.0999) ccw
  arc A472 (-27.7024, -17.1337) -> (-27.6909, -17.0137) centre (-27.7761, -17.0661) ccw
  arc A473 (-28.1198, -18.3355) -> (-27.0934, -18.0814) centre (-29.3655, -11.102) ccw
  arc A474 (-28.2207, -18.2913) -> (-28.1198, -18.3355) centre (-28.1367, -18.2369) ccw
  arc A475 (-26.0866, -19.384) -> (-26.2023, -19.3501) centre (-26.1669, -19.4436) ccw
  arc A476 (-27.4731, -19.2909) -> (-27.4696, -19.401) centre (-27.3879, -19.3433) ccw
  arc A477 (-26.8558, -18.4324) -> (-27.4731, -19.2909) centre (-21.2208, -23.1358) ccw
  arc A478 (-26.8558, -18.4324) -> (-26.85, -18.312) centre (-26.9326, -18.3684) ccw
  arc A479 (-27.2155, -19.6527) -> (-26.2023, -19.3501) centre (-28.804, -12.4866) ccw
  arc A480 (-27.3184, -19.6134) -> (-27.2155, -19.6527) centre (-27.2371, -19.5551) ccw
  arc A481 (-25.1348, -20.6033) -> (-25.2519, -20.5749) centre (-25.2121, -20.6666) ccw
  arc A482 (-26.5241, -20.5763) -> (-26.5154, -20.686) centre (-26.4365, -20.6245) ccw
  arc A483 (-25.9483, -19.6894) -> (-26.5241, -20.5763) centre (-20.0959, -24.1194) ccw
  arc A484 (-25.9483, -19.6894) -> (-25.9482, -19.5688) centre (-26.0281, -19.6291) ccw
  arc A485 (-26.2495, -20.9254) -> (-25.2519, -20.5749) centre (-28.1772, -13.8431) ccw
  arc A486 (-26.3542, -20.891) -> (-26.2495, -20.9254) centre (-26.2758, -20.8289) ccw
  arc A487 (-24.1259, -21.7759) -> (-24.2444, -21.7532) centre (-24.2002, -21.8429) ccw
  arc A488 (-25.515, -21.815) -> (-25.5011, -21.9243) centre (-25.4252, -21.8591) ccw
  arc A489 (-24.9821, -20.9018) -> (-25.515, -21.815) centre (-18.9255, -25.0482) ccw
  arc A490 (-24.9821, -20.9018) -> (-24.9877, -20.7813) centre (-25.0646, -20.8453) ccw
  arc A491 (-25.2241, -22.1507) -> (-24.2444, -21.7532) centre (-27.4867, -15.1681) ccw
  arc A492 (-25.3303, -22.1213) -> (-25.2241, -22.1507) centre (-25.255, -22.0556) ccw
  arc A493 (-23.0625, -22.8992) -> (-23.1818, -22.8821) centre (-23.1334, -22.9696) ccw
  arc A494 (-24.4481, -23.0044) -> (-24.429, -23.1128) centre (-24.3563, -23.0441) ccw
  arc A495 (-23.9592, -22.0668) -> (-24.4481, -23.0044) centre (-17.7122, -25.9204) ccw
  arc A496 (-23.9592, -22.0668) -> (-23.9706, -21.9468) centre (-24.0443, -22.0143) ccw
  arc A497 (-24.1416, -23.3258) -> (-23.1818, -22.8821) centre (-26.7338, -16.4588) ccw
  arc A498 (-24.249, -23.3015) -> (-24.1416, -23.3258) centre (-24.1769, -23.2323) ccw
  arc A499 (-21.9468, -23.9706) -> (-22.0668, -23.9592) centre (-22.0143, -24.0443) ccw
  arc A500 (-23.3258, -24.1416) -> (-23.3015, -24.249) centre (-23.2323, -24.1769) ccw
  arc A501 (-22.8821, -23.1818) -> (-23.3258, -24.1416) centre (-16.4588, -26.7338) ccw
  arc A502 (-22.8821, -23.1818) -> (-22.8992, -23.0625) centre (-22.9696, -23.1334) ccw
  arc A503 (-23.0044, -24.4481) -> (-22.0668, -23.9592) centre (-25.9204, -17.7122) ccw
  arc A504 (-23.1128, -24.429) -> (-23.0044, -24.4481) centre (-23.0441, -24.3563) ccw
  arc A505 (-20.7813, -24.9877) -> (-20.9018, -24.9821) centre (-20.8453, -25.0646) ccw
  arc A506 (-22.1507, -25.2241) -> (-22.1213, -25.3303) centre (-22.0556, -25.255) ccw
  arc A507 (-21.7532, -24.2444) -> (-22.1507, -25.2241) centre (-15.1681, -27.4867) ccw
  arc A508 (-21.7532, -24.2444) -> (-21.7759, -24.1259) centre (-21.8429, -24.2002) ccw
  arc A509 (-21.815, -25.515) -> (-20.9018, -24.9821) centre (-25.0482, -18.9255) ccw
  arc A510 (-21.9243, -25.5011) -> (-21.815, -25.515) centre (-21.8591, -25.4252) ccw
  arc A511 (-19.5688, -25.9482) -> (-19.6894, -25.9483) centre (-19.6291, -26.0281) ccw
  arc A512 (-20.9254, -26.2495) -> (-20.891, -26.3542) centre (-20.8289, -26.2758) ccw
  arc A513 (-20.5749, -25.2519) -> (-20.9254, -26.2495) centre (-13.8431, -28.1772) ccw
  arc A514 (-20.5749, -25.2519) -> (-20.6033, -25.1348) centre (-20.6666, -25.2121) ccw
  arc A515 (-20.5763, -26.5241) -> (-19.6894, -25.9483) centre (-24.1194, -20.0959) ccw
  arc A516 (-20.686, -26.5154) -> (-20.5763, -26.5241) centre (-20.6245, -26.4365) ccw
  arc A517 (-18.312, -26.85) -> (-18.4324, -26.8558) centre (-18.3684, -26.9326) ccw
  arc A518 (-19.6527, -27.2155) -> (-19.6134, -27.3184) centre (-19.5551, -27.2371) ccw
  arc A519 (-19.3501, -26.2023) -> (-19.6527, -27.2155) centre (-12.4866, -28.804) ccw
  arc A520 (-19.3501, -26.2023) -> (-19.384, -26.0866) centre (-19.4436, -26.1669) ccw
  arc A521 (-19.2909, -27.4731) -> (-18.4324, -26.8558) centre (-23.1358, -21.2208) ccw
  arc A522 (-19.401, -27.4696) -> (-19.2909, -27.4731) centre (-19.3433, -27.3879) ccw
  arc A523 (-17.0137, -27.6909) -> (-17.1337, -27.7024) centre (-17.0661, -27.7761) ccw
  arc A524 (-18.3355, -28.1198) -> (-18.2913, -28.2207) centre (-18.2369, -28.1367) ccw
  arc A525 (-18.0814, -27.0934) -> (-18.3355, -28.1198) centre (-11.102, -29.3655) ccw
  arc A526 (-18.0814, -27.0934) -> (-18.1207, -26.9794) centre (-18.1765, -27.0624) ccw
  arc A527 (-17.9618, -28.3599) -> (-17.1337, -27.7024) centre (-22.0999, -22.2976) ccw
  arc A528 (-18.0719, -28.3616) -> (-17.9618, -28.3599) centre (-18.0182, -28.2773) ccw
  arc A529 (-15.6768, -28.469) -> (-15.7962, -28.4863) centre (-15.7251, -28.5566) ccw
  arc A530 (-16.9767, -28.9603) -> (-16.9278, -29.059) centre (-16.8775, -28.9726) ccw
  arc A531 (-16.7718, -27.923) -> (-16.9767, -28.9603) centre (-9.6921, -29.8605) ccw
  arc A532 (-16.7718, -27.923) -> (-16.8165, -27.8111) centre (-16.8682, -27.8966) ccw
  arc A533 (-16.592, -29.1824) -> (-15.7962, -28.4863) centre (-21.0139, -23.3239) ccw
  arc A534 (-16.702, -29.1894) -> (-16.592, -29.1824) centre (-16.6523, -29.1026) ccw
  arc A535 (-14.3045, -29.1827) -> (-14.4228, -29.2057) centre (-14.3485, -29.2725) ccw
  arc A536 (-15.5795, -29.7353) -> (-15.5259, -29.8316) centre (-15.4798, -29.7429) ccw
  arc A537 (-15.4242, -28.6894) -> (-15.5795, -29.7353) centre (-8.2603, -30.2879) ccw
  arc A538 (-15.4242, -28.6894) -> (-15.4741, -28.5797) centre (-15.5218, -28.6677) ccw
  arc A539 (-15.1847, -29.9389) -> (-14.4228, -29.2057) centre (-19.8803, -24.2973) ccw
  arc A540 (-15.2941, -29.9511) -> (-15.1847, -29.9389) centre (-15.2487, -29.862) ccw
  arc A541 (-12.8997, -29.8303) -> (-13.0168, -29.8588) centre (-12.9394, -29.9221) ccw
  arc A542 (-14.147, -30.443) -> (-14.0889, -30.5365) centre (-14.047, -30.4457) ccw
  arc A543 (-14.0416, -29.3909) -> (-14.147, -30.443) centre (-6.8098, -30.6466) ccw
  arc A544 (-14.0416, -29.3909) -> (-14.0967, -29.2836) centre (-14.1401, -29.3738) ccw
  arc A545 (-13.743, -30.6275) -> (-13.0168, -29.8588) centre (-18.7017, -25.2158) ccw
  arc A546 (-13.8517, -30.6449) -> (-13.743, -30.6275) centre (-13.8105, -30.5537) ccw
  arc A547 (-11.4657, -30.4103) -> (-11.5814, -30.4444) centre (-11.501, -30.5039) ccw
  arc A548 (-12.6824, -31.0816) -> (-12.62, -31.1723) centre (-12.5824, -31.0796) ccw
  arc A549 (-12.6272, -30.0257) -> (-12.6824, -31.0816) centre (-5.3439, -30.9359) ccw
  arc A550 (-12.6272, -30.0257) -> (-12.6874, -29.9212) centre (-12.7264, -30.0133) ccw
  arc A551 (-12.2701, -31.2467) -> (-11.5814, -30.4444) centre (-17.4807, -26.0771) ccw
  arc A552 (-12.3779, -31.2692) -> (-12.2701, -31.2467) centre (-12.3411, -31.1763) ccw
  arc A553 (-10.0057, -30.9214) -> (-10.1196, -30.961) centre (-10.0365, -31.0166) ccw
  arc A554 (-11.1891, -31.6499) -> (-11.1224, -31.7375) centre (-11.0894, -31.6431) ccw
  arc A555 (-11.1842, -30.5925) -> (-11.1891, -31.6499) centre (-3.8658, -31.1551) ccw
  arc A556 (-11.1842, -30.5925) -> (-11.2493, -30.491) centre (-11.2839, -30.5848) ccw
  arc A557 (-10.7694, -31.7951) -> (-10.1196, -30.961) centre (-16.2201, -26.8793) ccw
  arc A558 (-10.876, -31.8228) -> (-10.7694, -31.7951) centre (-10.8437, -31.7282) ccw
  arc A559 (-8.5231, -31.3625) -> (-8.635, -31.4074) centre (-8.5493, -31.459) ccw
  arc A560 (-9.6705, -32.1464) -> (-9.5997, -32.2308) centre (-9.5712, -32.1349) ccw
  arc A561 (-9.7159, -31.09) -> (-9.6705, -32.1464) centre (-2.379, -31.3038) ccw
  arc A562 (-9.7159, -31.09) -> (-9.7858, -30.9918) centre (-9.8159, -31.0871) ccw
  arc A563 (-9.2443, -32.2715) -> (-8.635, -31.4074) centre (-14.9228, -27.6206) ccw
  arc A564 (-9.3495, -32.3042) -> (-9.2443, -32.2715) centre (-9.3217, -32.2082) ccw
  arc A565 (-7.0212, -31.7325) -> (-7.1308, -31.7827) centre (-7.0428, -31.8302) ccw
  arc A566 (-8.13, -32.5701) -> (-8.0552, -32.651) centre (-8.0313, -32.5539) ccw
  arc A567 (-8.2256, -31.5171) -> (-8.13, -32.5701) centre (-0.8868, -31.3815) ccw
  arc A568 (-8.2256, -31.5171) -> (-8.3, -31.4223) centre (-8.3256, -31.519) ccw
  arc A569 (-7.6983, -32.6749) -> (-7.1308, -31.7827) centre (-13.5916, -28.2994) ccw
  arc A570 (-7.8018, -32.7125) -> (-7.6983, -32.6749) centre (-7.7786, -32.6152) ccw
  arc A571 (-5.5033, -32.0307) -> (-5.6104, -32.086) centre (-5.5203, -32.1292) ccw
  arc A572 (-6.571, -32.9201) -> (-6.4925, -32.9973) centre (-6.4732, -32.8992) ccw
  arc A573 (-6.7166, -31.8728) -> (-6.571, -32.9201) centre (0.6074, -31.3882) ccw
  arc A574 (-6.7166, -31.8728) -> (-6.7955, -31.7816) centre (-6.8164, -31.8794) ccw
  arc A575 (-6.1349, -33.0041) -> (-5.6104, -32.086) centre (-12.2297, -28.9141) ccw
  arc A576 (-6.2364, -33.0467) -> (-6.1349, -33.0041) centre (-6.2179, -32.9484) ccw
  arc A577 (-3.973, -32.2562) -> (-4.0774, -32.3166) centre (-3.9852, -32.3555) ccw
  arc A578 (-4.9972, -33.1955) -> (-4.9151, -33.2689) centre (-4.9005, -33.17) ccw
  arc A579 (-5.1924, -32.1563) -> (-4.9972, -33.1955) centre (2.1002, -31.3237) ccw
  arc A580 (-5.1924, -32.1563) -> (-5.2756, -32.069) centre (-5.2918, -32.1676) ccw
  arc A581 (-4.5575, -33.2587) -> (-4.0774, -32.3166) centre (-10.84, -29.4632) ccw
  arc A582 (-4.657, -33.306) -> (-4.5575, -33.2587) centre (-4.6431, -33.207) ccw
  arc A583 (-2.4337, -32.4088) -> (-2.5351, -32.474) centre (-2.4412, -32.5085) ccw
  arc A584 (-3.412, -33.3956) -> (-3.3265, -33.4651) centre (-3.3166, -33.3656) ccw
  arc A585 (-3.6565, -32.3669) -> (-3.412, -33.3956) centre (3.5883, -31.1883) ccw
  arc A586 (-3.6565, -32.3669) -> (-3.7437, -32.2837) centre (-3.7552, -32.383) ccw
  arc A587 (-2.9698, -33.4379) -> (-2.5351, -32.474) centre (-9.4258, -29.9456) ccw
  arc A588 (-3.0669, -33.4899) -> (-2.9698, -33.4379) centre (-3.0578, -33.3903) ccw
  arc A589 (-0.8889, -32.4878) -> (-0.987, -32.5579) centre (-0.8916, -32.5878) ccw
  arc A590 (-1.8191, -33.5202) -> (-1.7304, -33.5855) centre (-1.7253, -33.4856) ccw
  arc A591 (-2.1123, -32.5043) -> (-1.8191, -33.5202) centre (5.0682, -30.9823) ccw
  arc A592 (-2.1123, -32.5043) -> (-2.2033, -32.4252) centre (-2.2101, -32.525) ccw
  arc A593 (-1.3754, -33.5413) -> (-0.987, -32.5579) centre (-7.9903, -30.3602) ccw
  arc A594 (-1.4699, -33.5979) -> (-1.3754, -33.5413) centre (-1.4656, -33.498) ccw